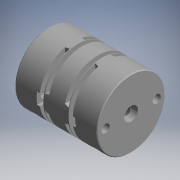
# Autodesk Inventor part: MCKL25-5-10_b
Saved by Autodesk Inventor 2017.3 (Build 213256000, 256)
## iProperties
Part Number: MCKL25-5-10_b
Material: Generic
Catalog Web Link: www.cadenas.de
Description: MCKL, MCKLLK, MCKLRK, MCKLWK_body-Disc Couplings - High Torque, Set Screw - Double Disc Type
Vendor: MISUMI
Document SubType Name: Modeling
Designer: partserver
Manufacturer: MISUMI
Mass: 10.3118 g
Surface Area: 70.129 cm^2
Volume: 10.3118 cm^3
Density: 1 g/cm^3
Appearance: PSOLRGB-192-192-192
Category: PARTsolutions
Company: MISUMI
Title: MCKL25-5-10
Author: Cadenas PARTsolutions
Comments: Disc Couplings - High Torque, Set Screw - Double Disc Type
PSOL_IDENT_0: {$CADENAS_DATA\23d-libs\misumi\metric\50_couplings\mckl\mckl.prj},249 {VTYP=3D},{NB=MCKL25-5-10_b},{
PSOL_IDENT_1: LINA=MCKL25-5-10},{NN=MCKL, MCKLLK, MCKLRK, MCKLWK_body},{DATE=30.06.2021 13:24:46},{GEOMDATE=08.10.
PSOL_IDENT_2: 2015 07:37:00},{VERSION=},{LINEID=80},{WBVAR=HS,KGHS,ALT1,DD1,LDC,ALT2,DD2,RDC,ALT3,ALT4},{WBNUMERIC=
PSOL_IDENT_3: DD1,LDC,DD2,RDC}  {NB=MCKL25-5-10_b},{LINA=MCKL25-5-10},{KT=DUMMY},{PN=MCKL25-5-10},{TYPE=MCKL},{HS=
PSOL_IDENT_4: },{HSALG= '','Standard Hole','KGH','Key Groove Hole' },{KGHS=},{KGHSALG= '','N/A' },{D=25},{DPN=25},
PSOL_IDENT_5: {ALT1=},{ALT1ALG= '','w/o LDC (Shaft Bore Dia. (Left Shaft))','LDC','with LDC (Shaft Bore Dia. (Left
PSOL_IDENT_6: Shaft))' },{DD1=5.00},{DD1ALG=[5,6,6.35,7,8,9.53,10,11,12]},{LDC=0.00},{LDCALG=[0]},{DD1PN=-5},{DD1
PSOL_IDENT_7: LDC=5.000},{ALT2=},{ALT2ALG= '','w/o RDC (Shaft Bore Dia. (Right Shaft))','RDC','with RDC (Shaft Bor
PSOL_IDENT_8: e Dia. (Right Shaft))' },{DD2=10.00},{DD2ALG=[5,6,6.35,7,8,9.53,10,11,12]},{RDC=0.00},{RDCALG=[0]},{
PSOL_IDENT_9: DD2PN=-10},{DD2RDC=10.000},{DD3=10.4},{L=30.2},{LL=9.0},{F=4.0},{M=M4},{ALT3=},{ALT3ALG= '','N/A' },
PSOL_IDENT_10: {KLH=0},{BBL=0},{TTL=0.0},{ALT3PN=},{KEYL=0.000},{ALT4=},{ALT4ALG= '','N/A' },{KRH=0},{BBR=0},{TTR=0
PSOL_IDENT_11: .0},{ALT4PN=},{KEYR=0.000},{HUBT=4.200},{HUBD=3.000},{HUBL=1.000},{PCD=18.800},{ATAW=9.750},{ATAH=11
PSOL_IDENT_12: .750},{ATAR=12.500},{ATAD=6.688},{ATAT=1.475},{ATADEG=14.000},{DISKD=12.000},{DISKT=0.250},{BOLTD=3.
PSOL_IDENT_13: 000},{BOLTH=1.000},{SPCL=5.800},{M3D=4.000},{ML3D=6.000},{LML1=10.000},{LML2=10.000},{RML1=7.500},{R
PSOL_IDENT_14: ML2=7.500},{CP1=2.500},{CP2=2.500},{CP3=5.000},{CP4=5.000}
NB: MCKL25-5-10_b
NN: MCKL, MCKLLK, MCKLRK, MCKLWK_body
NT: Disc Couplings - High Torque, Set Screw - Double Disc Type
NBSYN: $PN._b
LINA: MCKL25-5-10
CATALOG: Misumi
PN: MCKL25-5-10
HS: Standard Hole
KGHS: N/A
D: 25
ALT1: w/o LDC (Shaft Bore Dia. (Left Shaft))
DD1: 5
LDC: 0
ALT2: w/o RDC (Shaft Bore Dia. (Right Shaft))
DD2: 10
RDC: 0
DD3: 10.4
L: 30.2
LL: 9
F: 4
M: M4
ALT3: N/A
KLH: 0
BBL: 0
TTL: 0
ALT4: N/A
KRH: 0
BBR: 0
TTR: 0
HUBT: 4.2
HUBD: 3
HUBL: 1
PCD: 18.8
ATAW: 9.75
ATAH: 11.75
ATAR: 12.5
ATAD: 6.688
ATAT: 1.475
ATADEG: 14
DISKD: 12
DISKT: 0.25
BOLTD: 3
BOLTH: 1
SPCL: 5.8
SUPPLIER: MISUMI
ARTICLENO: MCKL25-5-10_b
BOMINFO: MCKL25-5-10
CREATOR: CADENAS GmbH
Autodesk Inventor part; units mm, degrees
sketch "Sketch_1" plane through (0, 0, 0) normal (0, 0, 1) x (1, 0, 0)
  line L0 (9, 0) -> (0, 0)
  line L1 (0, 0) -> (0, 15)
  line L2 (0, 15) -> (9, 15)
  line L3 (9, 15) -> (9, 0)
  line L4 (9, 0) -> (0, 0)
  constraints: 10 end point
revolve "Revolution1" add sketch "Sketch_1" angle 360 about axis through (9, 0, 0) along (1, 0, 0)
sketch "Sketch_65" plane through (0, 0, 0) normal (0, 0, 1) x (1, 0, 0)
  line L0 (10.475, 0) -> (0, 0)
  line L1 (0, 0) -> (0, 2.5)
  line L2 (0, 2.5) -> (10.475, 2.5)
  line L3 (10.475, 2.5) -> (10.475, 0)
  line L4 (10.475, 0) -> (0, 0)
  constraints: 10 end point
revolve "Revolution2" cut sketch "Sketch_65" angle 360 about axis through (10.475, 0, 0) along (1, 0, 0)
sketch "Sketch_2" plane through (10.475, 0, 0) normal (1, 0, 0) x (0, 0, -1)
  arc A0 (-14.8117, 2.3692) -> (-14.8117, -2.3692) centre (0, 0) ccw
  arc A1 (-14.8117, -2.3692) -> (-3.9278, 0) centre (-11.75, 9.75) ccw
  arc A2 (-3.9278, 0) -> (-14.8117, 2.3692) centre (-11.75, -9.75) ccw
  constraints: 6 point on circle, 3 centre point
extrude "Extrusion1" add sketch "Sketch_2" against normal blind 1.475 draft 14
sketch "_p_______1_SKETCH_1" plane through (10.475, 0, 0) normal (1, 0, 0) x (0, 0, -1)
  arc A0 (14.8117, -2.3692) -> (14.8117, 2.3692) centre (0, 0) ccw
  arc A1 (14.8117, 2.3692) -> (3.9278, 0) centre (11.75, -9.75) ccw
  arc A2 (3.9278, 0) -> (14.8117, -2.3692) centre (11.75, 9.75) ccw
  constraints: 6 point on circle, 3 centre point
extrude "Extrusion2" add sketch "_p_______1_SKETCH_1" against normal blind 1.475 draft 14
sketch "Sketch_15" plane through (10.475, 0, 0) normal (1, 0, 0) x (0, 0, -1)
  circle A0 centre (0, 0) radius 6.688
  constraints: 1 centre point
extrude "Extrusion3" cut sketch "Sketch_15" against normal blind 1.475 draft -14
sketch "Sketch_40" plane through (0, 0, 0) normal (0, 0, 1) x (1, 0, 0)
  line L0 (10.725, 0) -> (10.475, 0)
  line L1 (10.475, 0) -> (10.475, 15)
  line L2 (10.475, 15) -> (10.725, 15)
  line L3 (10.725, 15) -> (10.725, 0)
  line L4 (10.725, 0) -> (10.475, 0)
  constraints: 10 end point
revolve "Revolution3" add sketch "Sketch_40" angle 360 about axis through (10.725, 0, 0) along (1, 0, 0)
sketch "Sketch7" plane through (10.725, 0, 0) normal (1, 0, 0) x (0, 0, -1)
  point P0 (0, 0)
hole "Hole1" at (10.725, 0, 0) direction (-1, 0, 0) diameter 12 depth 0.25
sketch "Sketch_43" plane through (10.725, 0, 0) normal (1, 0, 0) x (0, 0, -1)
  arc A0 (-2.3692, 14.8117) -> (0, 3.9278) centre (9.75, 11.75) ccw
  arc A1 (0, 3.9278) -> (2.3692, 14.8117) centre (-9.75, 11.75) ccw
  arc A2 (2.3692, 14.8117) -> (-2.3692, 14.8117) centre (0, 0) ccw
  constraints: 6 point on circle, 3 centre point
extrude "Extrusion4" add sketch "Sketch_43" along normal blind 1.475 draft 14
sketch "_p_______2_SKETCH_1" plane through (10.725, 0, 0) normal (1, 0, 0) x (0, 0, -1)
  arc A0 (2.3692, -14.8117) -> (0, -3.9278) centre (-9.75, -11.75) ccw
  arc A1 (0, -3.9278) -> (-2.3692, -14.8117) centre (9.75, -11.75) ccw
  arc A2 (-2.3692, -14.8117) -> (2.3692, -14.8117) centre (0, 0) ccw
  constraints: 6 point on circle, 3 centre point
extrude "Extrusion5" add sketch "_p_______2_SKETCH_1" along normal blind 1.475 draft 14
sketch "Sketch_49" plane through (10.725, 0, 0) normal (1, 0, 0) x (0, 0, -1)
  circle A0 centre (0, 0) radius 6.688
  constraints: 1 centre point
extrude "Extrusion6" cut sketch "Sketch_49" along normal blind 1.475 draft -10
sketch "Sketch_48" plane through (0, 0, 0) normal (0, 0, 1) x (1, 0, 0)
  line L0 (18, 0) -> (12.2, 0)
  line L1 (12.2, 0) -> (12.2, 15)
  line L2 (12.2, 15) -> (18, 15)
  line L3 (18, 15) -> (18, 0)
  line L4 (18, 0) -> (12.2, 0)
  constraints: 10 end point
revolve "Revolution4" add sketch "Sketch_48" angle 360 about axis through (18, 0, 0) along (1, 0, 0)
sketch "Sketch_66" plane through (0, 0, 0) normal (0, 0, 1) x (1, 0, 0)
  line L0 (19.475, 0) -> (10.725, 0)
  line L1 (10.725, 0) -> (10.725, 5.2)
  line L2 (10.725, 5.2) -> (19.475, 5.2)
  line L3 (19.475, 5.2) -> (19.475, 0)
  line L4 (19.475, 0) -> (10.725, 0)
  constraints: 10 end point
revolve "Revolution5" cut sketch "Sketch_66" angle 360 about axis through (19.475, 0, 0) along (1, 0, 0)
sketch "Sketch_50" plane through (19.475, 0, 0) normal (1, 0, 0) x (0, 0, -1)
  arc A0 (-2.3692, 14.8117) -> (0, 3.9278) centre (9.75, 11.75) ccw
  arc A1 (0, 3.9278) -> (2.3692, 14.8117) centre (-9.75, 11.75) ccw
  arc A2 (2.3692, 14.8117) -> (-2.3692, 14.8117) centre (0, 0) ccw
  constraints: 6 point on circle, 3 centre point
extrude "Extrusion7" add sketch "Sketch_50" against normal blind 1.475 draft 14
sketch "_p_______3_SKETCH_1" plane through (19.475, 0, 0) normal (1, 0, 0) x (0, 0, -1)
  arc A0 (2.3692, -14.8117) -> (0, -3.9278) centre (-9.75, -11.75) ccw
  arc A1 (0, -3.9278) -> (-2.3692, -14.8117) centre (9.75, -11.75) ccw
  arc A2 (-2.3692, -14.8117) -> (2.3692, -14.8117) centre (0, 0) ccw
  constraints: 6 point on circle, 3 centre point
extrude "Extrusion8" add sketch "_p_______3_SKETCH_1" against normal blind 1.475 draft 14
sketch "Sketch_52" plane through (19.475, 0, 0) normal (1, 0, 0) x (0, 0, -1)
  circle A0 centre (0, 0) radius 6.688
  constraints: 1 centre point
extrude "Extrusion9" cut sketch "Sketch_52" against normal blind 1.475 draft -14
sketch "Sketch_53" plane through (0, 0, 0) normal (0, 0, 1) x (1, 0, 0)
  line L0 (19.725, 0) -> (19.475, 0)
  line L1 (19.475, 0) -> (19.475, 15)
  line L2 (19.475, 15) -> (19.725, 15)
  line L3 (19.725, 15) -> (19.725, 0)
  line L4 (19.725, 0) -> (19.475, 0)
  constraints: 10 end point
revolve "Revolution6" add sketch "Sketch_53" angle 360 about axis through (19.725, 0, 0) along (1, 0, 0)
sketch "Sketch17" plane through (19.725, 0, 0) normal (1, 0, 0) x (0, 0, -1)
  point P0 (0, 0)
hole "Hole2" at (19.725, 0, 0) direction (-1, 0, 0) diameter 12 depth 0.25
sketch "Sketch_54" plane through (19.725, 0, 0) normal (1, 0, 0) x (0, 0, -1)
  arc A0 (-14.8117, 2.3692) -> (-14.8117, -2.3692) centre (0, 0) ccw
  arc A1 (-14.8117, -2.3692) -> (-3.9278, 0) centre (-11.75, 9.75) ccw
  arc A2 (-3.9278, 0) -> (-14.8117, 2.3692) centre (-11.75, -9.75) ccw
  constraints: 6 point on circle, 3 centre point
extrude "Extrusion10" add sketch "Sketch_54" along normal blind 1.475 draft 14
sketch "_p_______4_SKETCH_1" plane through (19.725, 0, 0) normal (1, 0, 0) x (0, 0, -1)
  arc A0 (14.8117, -2.3692) -> (14.8117, 2.3692) centre (0, 0) ccw
  arc A1 (14.8117, 2.3692) -> (3.9278, 0) centre (11.75, -9.75) ccw
  arc A2 (3.9278, 0) -> (14.8117, -2.3692) centre (11.75, 9.75) ccw
  constraints: 6 point on circle, 3 centre point
extrude "Extrusion11" add sketch "_p_______4_SKETCH_1" along normal blind 1.475 draft 14
sketch "Sketch_56" plane through (19.725, 0, 0) normal (1, 0, 0) x (0, 0, -1)
  circle A0 centre (0, 0) radius 6.688
  constraints: 1 centre point
extrude "Extrusion12" cut sketch "Sketch_56" along normal blind 1.475 draft -14
sketch "Sketch_57" plane through (0, 0, 0) normal (0, 0, 1) x (1, 0, 0)
  line L0 (30.2, 0) -> (21.2, 0)
  line L1 (21.2, 0) -> (21.2, 15)
  line L2 (21.2, 15) -> (30.2, 15)
  line L3 (30.2, 15) -> (30.2, 0)
  line L4 (30.2, 0) -> (21.2, 0)
  constraints: 10 end point
revolve "Revolution7" add sketch "Sketch_57" angle 360 about axis through (30.2, 0, 0) along (1, 0, 0)
sketch "Sketch22" plane through (30.2, 0, 0) normal (1, 0, 0) x (0, 0, -1)
  point P0 (0, 0)
hole "Hole3" at (30.2, 0, 0) direction (-1, 0, 0) diameter 10 depth 10.475
sketch "Sketch_8" plane through (0, 0, 0) normal (0, 0, 1) x (1, 0, 0)
  line L0 (30.2, 0) -> (0, 0)
  line L1 (0, 25) -> (0, 12.25)
  line L2 (0, 12.25) -> (0.25, 12.5)
  line L3 (0.25, 12.5) -> (29.95, 12.5)
  line L4 (29.95, 12.5) -> (30.2, 12.25)
  line L5 (30.2, 12.25) -> (30.2, 25)
  line L6 (30.2, 25) -> (0, 25)
  constraints: 14 end point
revolve "Revolution8" cut sketch "Sketch_8" angle 360 about axis through (30.2, 0, 0) along (1, 0, 0)
sketch "Sketch24" plane through (9, 0, 0) normal (1, 0, 0) x (0, 0, -1)
  point P0 (0, 9.4)
hole "Hole4" at (9, 9.4, 0) direction (-1, 0, 0) diameter 3 depth 9
pattern_linear "Rectangular Pattern1" count 2 spacing 18.8 along (0, -1, 0) of "Hole4"
sketch "Sketch_59" plane through (9, 0, 0) normal (1, 0, 0) x (0, 0, -1)
  line L0 (-2.1, 12.3223) -> (-2.1, 9.4)
  arc A0 (-2.1, 9.4) -> (2.1, 9.4) centre (0, 9.4) ccw
  line L1 (2.1, 9.4) -> (2.1, 12.3223)
  arc A1 (2.1, 12.3223) -> (-2.1, 12.3223) centre (0, 0) ccw
  constraints: 4 end point, 4 point on circle, 2 centre point
extrude "Extrusion13" cut sketch "Sketch_59" against normal blind 1
sketch "_p_______6_SKETCH_1" plane through (9, 0, 0) normal (1, 0, 0) x (0, 0, -1)
  line L0 (2.1, -12.3223) -> (2.1, -9.4)
  arc A0 (2.1, -9.4) -> (-2.1, -9.4) centre (0, -9.4) ccw
  line L1 (-2.1, -9.4) -> (-2.1, -12.3223)
  arc A1 (-2.1, -12.3223) -> (2.1, -12.3223) centre (0, 0) ccw
  constraints: 4 end point, 4 point on circle, 2 centre point
extrude "Extrusion14" cut sketch "_p_______6_SKETCH_1" against normal blind 1
sketch "Sketch27" plane through (30.2, 0, 0) normal (1, 0, 0) x (0, 0, -1)
  point P0 (0, 9.4)
hole "Hole5" at (30.2, 9.4, 0) direction (-1, 0, 0) diameter 3 depth 9
pattern_linear "Rectangular Pattern2" count 2 spacing 18.8 along (0, -1, 0) of "Hole5"
sketch "Sketch_72" plane through (21.2, 0, 0) normal (1, 0, 0) x (0, 0, -1)
  line L0 (-2.1, 12.3223) -> (-2.1, 9.4)
  arc A0 (-2.1, 9.4) -> (2.1, 9.4) centre (0, 9.4) ccw
  line L1 (2.1, 9.4) -> (2.1, 12.3223)
  arc A1 (2.1, 12.3223) -> (-2.1, 12.3223) centre (0, 0) ccw
  constraints: 4 end point, 4 point on circle, 2 centre point
extrude "Extrusion15" cut sketch "Sketch_72" along normal blind 1
sketch "_p_______8_SKETCH_1" plane through (21.2, 0, 0) normal (1, 0, 0) x (0, 0, -1)
  line L0 (2.1, -12.3223) -> (2.1, -9.4)
  arc A0 (2.1, -9.4) -> (-2.1, -9.4) centre (0, -9.4) ccw
  line L1 (-2.1, -9.4) -> (-2.1, -12.3223)
  arc A1 (-2.1, -12.3223) -> (2.1, -12.3223) centre (0, 0) ccw
  constraints: 4 end point, 4 point on circle, 2 centre point
extrude "Extrusion16" cut sketch "_p_______8_SKETCH_1" along normal blind 1
sketch "Sketch_5" plane through (0, 0, 0) normal (0, 0, 1) x (1, 0, 0)
  line L0 (10.475, 9.4) -> (9.475, 9.4)
  line L1 (9.475, 9.4) -> (9.475, 10.9)
  line L2 (9.475, 10.9) -> (10.475, 10.9)
  line L3 (10.475, 10.9) -> (10.475, 9.4)
  line L4 (10.475, 9.4) -> (9.475, 9.4)
  constraints: 10 end point
revolve "Revolution9" add sketch "Sketch_5" angle 360 about axis through (10.475, 9.4, 0) along (1, 0, 0)
pattern_linear "Rectangular Pattern3" count 2 spacing 18.8 along (0, -1, 0) of "Revolution9"
sketch "Sketch_18" plane through (0, 0, 0) normal (0, 1, 0) x (1, 0, 0)
  line L0 (11.725, 9.4) -> (10.725, 9.4)
  line L1 (10.725, 9.4) -> (10.725, 10.9)
  line L2 (10.725, 10.9) -> (11.725, 10.9)
  line L3 (11.725, 10.9) -> (11.725, 9.4)
  line L4 (11.725, 9.4) -> (10.725, 9.4)
  constraints: 10 end point
revolve "Revolution10" add sketch "Sketch_18" angle 360 about axis through (11.725, 0, -9.4) along (1, 0, 0)
pattern_linear "Rectangular Pattern4" count 2 spacing 18.8 along (0, 0, 1) of "Revolution10"
sketch "Sketch_20" plane through (0, 0, 0) normal (0, 0, 1) x (1, 0, 0)
  line L0 (20.725, 9.4) -> (19.725, 9.4)
  line L1 (19.725, 9.4) -> (19.725, 10.9)
  line L2 (19.725, 10.9) -> (20.725, 10.9)
  line L3 (20.725, 10.9) -> (20.725, 9.4)
  line L4 (20.725, 9.4) -> (19.725, 9.4)
  constraints: 10 end point
revolve "Revolution11" add sketch "Sketch_20" angle 360 about axis through (20.725, 9.4, 0) along (1, 0, 0)
pattern_linear "Rectangular Pattern5" count 2 spacing 18.8 along (0, -1, 0) of "Revolution11"
sketch "Sketch_22" plane through (0, 0, 0) normal (0, 1, 0) x (1, 0, 0)
  line L0 (19.475, 9.4) -> (18.475, 9.4)
  line L1 (18.475, 9.4) -> (18.475, 10.9)
  line L2 (18.475, 10.9) -> (19.475, 10.9)
  line L3 (19.475, 10.9) -> (19.475, 9.4)
  line L4 (19.475, 9.4) -> (18.475, 9.4)
  constraints: 10 end point
revolve "Revolution12" add sketch "Sketch_22" angle 360 about axis through (19.475, 0, -9.4) along (1, 0, 0)
pattern_linear "Rectangular Pattern6" count 2 spacing 18.8 along (0, 0, 1) of "Revolution12"
sketch "Sketch_34" plane through (4, 0, 0) normal (1, 0, 0) x (0, 0, -1)
  line L0 (0, 0) -> (-8.8388, 8.8388)
  line L1 (-8.8388, 8.8388) -> (-7.4246, 10.253)
  line L2 (-7.4246, 10.253) -> (-7.4246, 9.7171)
  line L3 (-7.4246, 9.7171) -> (1.1462, 1.1462)
  line L4 (1.1462, 1.1462) -> (0, 0)
  line L5 (0, 0) -> (-8.8388, 8.8388)
  constraints: 12 end point
revolve "Revolution13" cut sketch "Sketch_34" angle 360 about axis through (4, 0, 0) along (0, -0.7071068, -0.7071068)
thread "Thread1" size "M4x0.7" class "6H" standard "ISO Metric profile" length 9.621
sketch "Sketch_3" plane through (4, 0, 0) normal (1, 0, 0) x (0, 0, -1)
  line L0 (0, 0) -> (-8.8388, -8.8388)
  line L1 (-8.8388, -8.8388) -> (-10.253, -7.4246)
  line L2 (-10.253, -7.4246) -> (-9.7171, -7.4246)
  line L3 (-9.7171, -7.4246) -> (-1.1462, 1.1462)
  line L4 (-1.1462, 1.1462) -> (0, 0)
  line L5 (0, 0) -> (-8.8388, -8.8388)
  constraints: 12 end point
revolve "Revolution14" cut sketch "Sketch_3" angle 360 about axis through (4, 0, 0) along (0, 0.7071068, -0.7071068)
thread "Thread2" size "M4x0.7" class "6H" standard "ISO Metric profile" length 9.621
sketch "Sketch_7" plane through (26.2, 0, 0) normal (1, 0, 0) x (0, 0, -1)
  line L0 (0, 0) -> (-8.8388, 8.8388)
  line L1 (-8.8388, 8.8388) -> (-7.4246, 10.253)
  line L2 (-7.4246, 10.253) -> (-7.4246, 9.7171)
  line L3 (-7.4246, 9.7171) -> (1.1462, 1.1462)
  line L4 (1.1462, 1.1462) -> (0, 0)
  line L5 (0, 0) -> (-8.8388, 8.8388)
  constraints: 12 end point
revolve "Revolution15" cut sketch "Sketch_7" angle 360 about axis through (26.2, 0, 0) along (0, -0.7071068, -0.7071068)
thread "Thread3" size "M4x0.7" class "6H" standard "ISO Metric profile" full length
sketch "Sketch_4" plane through (26.2, 0, 0) normal (1, 0, 0) x (0, 0, -1)
  line L0 (0, 0) -> (-8.8388, -8.8388)
  line L1 (-8.8388, -8.8388) -> (-10.253, -7.4246)
  line L2 (-10.253, -7.4246) -> (-9.7171, -7.4246)
  line L3 (-9.7171, -7.4246) -> (-1.1462, 1.1462)
  line L4 (-1.1462, 1.1462) -> (0, 0)
  line L5 (0, 0) -> (-8.8388, -8.8388)
  constraints: 12 end point
revolve "Revolution16" cut sketch "Sketch_4" angle 360 about axis through (26.2, 0, 0) along (0, 0.7071068, -0.7071068)
thread "Thread4" size "M4x0.7" class "6H" standard "ISO Metric profile" full length
ref_plane "to_set_screw1_XY" through (4, -1.7678, 1.7678) normal (0, -0.7071068, 0.7071068) x (1, 0, 0)
ref_plane "to_set_screw1_YZ" through (4, -1.7678, 1.7678) normal (1, 0, 0) x (0, 0.7071068, 0.7071068)
ref_plane "to_set_screw1_ZX" through (4, -1.7678, 1.7678) normal (0, 0.7071068, 0.7071068) x (0, -0.7071068, 0.7071068)
ref_plane "to_set_screw2_XY" through (4, 1.7678, 1.7678) normal (0, 0.7071068, 0.7071068) x (1, 0, 0)
ref_plane "to_set_screw2_YZ" through (4, 1.7678, 1.7678) normal (1, 0, 0) x (0, 0.7071068, -0.7071068)
ref_plane "to_set_screw2_ZX" through (4, 1.7678, 1.7678) normal (0, 0.7071068, -0.7071068) x (0, 0.7071068, 0.7071068)
ref_plane "to_set_screw3_XY" through (26.2, 3.5355, 3.5355) normal (0, 0.7071068, 0.7071068) x (1, 0, 0)
ref_plane "to_set_screw3_YZ" through (26.2, 3.5355, 3.5355) normal (1, 0, 0) x (0, 0.7071068, -0.7071068)
ref_plane "to_set_screw3_ZX" through (26.2, 3.5355, 3.5355) normal (0, 0.7071068, -0.7071068) x (0, 0.7071068, 0.7071068)
ref_plane "to_set_screw4_XY" through (26.2, -3.5355, 3.5355) normal (0, -0.7071068, 0.7071068) x (1, 0, 0)
ref_plane "to_set_screw4_YZ" through (26.2, -3.5355, 3.5355) normal (1, 0, 0) x (0, 0.7071068, 0.7071068)
ref_plane "to_set_screw4_ZX" through (26.2, -3.5355, 3.5355) normal (0, 0.7071068, 0.7071068) x (0, -0.7071068, 0.7071068)
body "Solid1"
